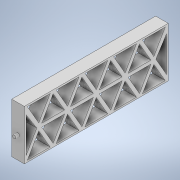
# Autodesk Inventor part: Arm support for middle arms
Saved by Autodesk Inventor 2020.2 (Build 242310000, 310)
## iProperties
Created: 2020-03-31
Part Number: Arm support for middle arms
Material: Generic
Document SubType Name: Modeling
Designer: Amaan Khalid
Density: 1 g/cm^3
Appearance: Default
Author: Amaan Khalid
Autodesk Inventor part; units mm, degrees
ref_plane "YZ Plane" through (0, 0, 0) normal (1, 0, 0) x (0, 1, 0)
ref_plane "XZ Plane" through (0, 0, 0) normal (0, 1, 0) x (-1, 0, 0)
ref_plane "XY Plane" through (0, 0, 0) normal (0, 0, 1) x (1, 0, 0)
sketch "Sketch1" plane through (0, 0, 0) normal (1, 0, 0) x (0, 1, 0)
  line L0 (33.6396, 9.7397) -> (33.6396, -13.1356)
  line L1 (33.6396, -13.1356) -> (53.4502, -1.698)
  line L2 (53.4502, -1.698) -> (33.6396, 9.7397)
  line L3 (50.707, -1.698) -> (35.0112, -10.7599)
  line L4 (35.0112, -10.7599) -> (35.0112, 7.364)
  line L5 (35.0112, 7.364) -> (50.707, -1.698)
  line L6 (53.4502, -1.698) -> (33.6396, -13.1356)
  line L7 (53.4502, -24.5732) -> (33.6396, -13.1356)
  line L8 (53.4502, -1.698) -> (53.4502, -24.5732)
  line L9 (52.0786, -4.0736) -> (36.3828, -13.1356)
  line L10 (36.3828, -13.1356) -> (52.0786, -22.1975)
  line L11 (52.0786, -22.1975) -> (52.0786, -4.0736)
  line L12 (33.6396, -13.1356) -> (33.6396, -36.0108)
  line L13 (33.6396, -36.0108) -> (53.4502, -24.5732)
  line L14 (35.0112, -33.6351) -> (35.0112, -15.5113)
  line L15 (35.0112, -15.5113) -> (50.707, -24.5732)
  line L16 (50.707, -24.5732) -> (35.0112, -33.6351)
  line L17 (53.4502, -24.5732) -> (53.4502, -47.4484)
  line L18 (53.4502, -47.4484) -> (33.6396, -36.0108)
  line L19 (52.0786, -45.0728) -> (52.0786, -26.9489)
  line L20 (36.3828, -36.0108) -> (52.0786, -45.0728)
  line L21 (52.0786, -26.9489) -> (36.3828, -36.0108)
  line L22 (33.6396, -36.0108) -> (33.6396, -58.8861)
  line L23 (35.0112, -56.5104) -> (35.0112, -38.3865)
  line L24 (33.6396, -58.8861) -> (53.4502, -47.4484)
  line L25 (50.707, -47.4484) -> (35.0112, -56.5104)
  line L26 (35.0112, -38.3865) -> (50.707, -47.4484)
  line L27 (53.4502, -47.4484) -> (53.4502, -70.3237)
  line L28 (52.0786, -49.8241) -> (36.3828, -58.8861)
  line L29 (36.3828, -58.8861) -> (52.0786, -67.948)
  line L30 (53.4502, -70.3237) -> (33.6396, -58.8861)
  line L31 (52.0786, -67.948) -> (52.0786, -49.8241)
  line L32 (33.6396, -58.8861) -> (33.6396, -81.7613)
  line L33 (33.6396, -81.7613) -> (53.4502, -70.3237)
  line L34 (50.707, -70.3237) -> (35.0112, -79.3856)
  line L35 (35.0112, -79.3856) -> (35.0112, -61.2617)
  line L36 (35.0112, -61.2617) -> (50.707, -70.3237)
  line L37 (33.6396, -13.1356) -> (13.8291, -1.698)
  line L38 (13.8291, -1.698) -> (33.6396, 9.7397)
  line L39 (16.5723, -1.698) -> (32.268, -10.7599)
  line L40 (32.268, -10.7599) -> (32.268, 7.364)
  line L41 (32.268, 7.364) -> (16.5723, -1.698)
  line L42 (33.6396, -13.1356) -> (13.8291, -1.698)
  line L43 (13.8291, -24.5732) -> (33.6396, -13.1356)
  line L44 (13.8291, -1.698) -> (13.8291, -24.5732)
  line L45 (15.2007, -4.0736) -> (30.8964, -13.1356)
  line L46 (30.8964, -13.1356) -> (15.2007, -22.1975)
  line L47 (15.2007, -22.1975) -> (15.2007, -4.0736)
  line L48 (13.8291, -24.5732) -> (33.6396, -13.1356)
  line L49 (33.6396, -36.0108) -> (13.8291, -24.5732)
  line L50 (32.268, -15.5113) -> (16.5723, -24.5732)
  line L51 (32.268, -33.6351) -> (32.268, -15.5113)
  line L52 (16.5723, -24.5732) -> (32.268, -33.6351)
  line L53 (13.8291, -47.4484) -> (33.6396, -36.0108)
  line L54 (16.5723, -47.4484) -> (32.268, -56.5104)
  line L55 (32.268, -56.5104) -> (32.268, -38.3865)
  line L56 (33.6396, -58.8861) -> (13.8291, -47.4484)
  line L57 (32.268, -38.3865) -> (16.5723, -47.4484)
  line L58 (33.6396, -36.0108) -> (13.8291, -24.5732)
  line L59 (15.2007, -26.9489) -> (30.8964, -36.0108)
  line L60 (13.8291, -24.5732) -> (13.8291, -47.4484)
  line L61 (15.2007, -45.0728) -> (15.2007, -26.9489)
  line L62 (13.8291, -47.4484) -> (33.6396, -36.0108)
  line L63 (30.8964, -36.0108) -> (15.2007, -45.0728)
  line L64 (13.8291, -70.3237) -> (33.6396, -58.8861)
  line L65 (32.268, -79.3856) -> (32.268, -61.2617)
  line L66 (33.6396, -81.7613) -> (13.8291, -70.3237)
  line L67 (32.268, -61.2617) -> (16.5723, -70.3237)
  line L68 (16.5723, -70.3237) -> (32.268, -79.3856)
  line L69 (33.6396, -58.8861) -> (13.8291, -47.4484)
  line L70 (13.8291, -47.4484) -> (13.8291, -70.3237)
  line L71 (15.2007, -67.948) -> (15.2007, -49.8241)
  line L72 (15.2007, -49.8241) -> (30.8964, -58.8861)
  line L73 (13.8291, -70.3237) -> (33.6396, -58.8861)
  line L74 (30.8964, -58.8861) -> (15.2007, -67.948)
  line L75 (13.8291, -1.698) -> (13.8291, 21.1773)
  line L76 (13.8291, 21.1773) -> (33.6396, 9.7397)
  line L77 (53.4502, -1.698) -> (53.4502, 21.1773)
  line L78 (53.4502, 21.1773) -> (33.6396, 9.7397)
  line L79 (53.4502, 21.1773) -> (13.8291, 21.1773)
  line L80 (53.4502, -70.3237) -> (53.4502, -93.1989)
  line L81 (53.4502, -93.1989) -> (33.6396, -81.7613)
  line L82 (13.8291, -70.3237) -> (13.8291, -93.1989)
  line L83 (13.8291, -93.1989) -> (33.6396, -81.7613)
  line L84 (53.4502, -93.1989) -> (13.8291, -93.1989)
  line L85 (15.2007, 0.6777) -> (15.2007, 18.8016)
  line L86 (30.8964, 9.7397) -> (15.2007, 0.6777)
  line L87 (15.2007, 18.8016) -> (30.8964, 9.7397)
  line L88 (52.0786, 0.6777) -> (52.0786, 18.8016)
  line L89 (52.0786, 18.8016) -> (36.3828, 9.7397)
  line L90 (36.3828, 9.7397) -> (52.0786, 0.6777)
  line L91 (36.3828, -81.7613) -> (52.0786, -90.8232)
  line L92 (52.0786, -90.8232) -> (52.0786, -72.6994)
  line L93 (52.0786, -72.6994) -> (36.3828, -81.7613)
  line L94 (30.8964, -81.7613) -> (15.2007, -90.8232)
  line L95 (15.2007, -90.8232) -> (15.2007, -72.6994)
  line L96 (15.2007, -72.6994) -> (30.8964, -81.7613)
  line L97 (35.8485, 19.8048) -> (46.9126, 19.8048)
  line L98 (46.9126, 19.8048) -> (33.6396, 11.3245)
  line L99 (33.6396, 11.3245) -> (18.9514, 19.8048)
  line L100 (18.9514, 19.8048) -> (35.8485, 19.8048)
  line L101 (35.8485, -91.8264) -> (46.9126, -91.8264)
  line L102 (46.9126, -91.8264) -> (33.6396, -83.3461)
  line L103 (33.6396, -83.3461) -> (18.9514, -91.8264)
  line L104 (18.9514, -91.8264) -> (35.8485, -91.8264)
  dimension "d13" = 1.3716
  constraints: 210 end point, 61 symmetric about line, 5 vertical, 3 collinear, 2 point on line, 1 parallel, 2 other
  measures "d13" distance between parallel lines of L1 L3
extrude "Extrusion1" add sketch "Sketch1" along normal blind 10
sketch "Sketch2" plane through (0, 13.8291, 21.1773) normal (0, 0, 1) x (1, 0, 0)
  line L0 (0, 39.6211) -> (10, 39.6211) projected
  circle A0 centre (5.0038, 17.6108) radius 1.27
  point P0 (0, -13.8291)
  point P1 (0, 19.8105)
  constraints: 1 centre point
extrude "Extrusion2" add sketch "Sketch2" along normal blind 3
sketch "Sketch3" plane through (0, 13.8291, -93.1989) normal (0, 0, -1) x (-1, 0, 0)
  line L0 (0, 39.6211) -> (-10, 39.6211) projected
  line L1 (0, 21.1821) -> (-10, 21.1821) projected
  circle A0 centre (-5, 21.1821) radius 1.27
  point P0 (0, -13.8291)
  dimension "d36" = 2.54
  constraints: 1 centre point, 1 midpoint
  measures "d36" diameter of A0
extrude "Extrusion3" add sketch "Sketch3" along normal blind 3
body "Solid1"
